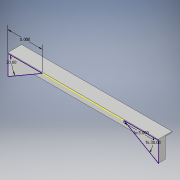
# Autodesk Inventor part: Wire Housing Lid vglue
Saved by Autodesk Inventor 2019 (Build 230136000, 136)
## iProperties
Created: 2020-03-05
Part Number: Wire Housing Lid vglue
Material: Generic
Document SubType Name: Modeling
Designer: Obscure_Decision
Density: 1 g/cm^3
Appearance: Default
Author: Obscure_Decision
Autodesk Inventor part; units mm, degrees
ref_plane "YZ Plane" through (0, 0, 0) normal (1, 0, 0) x (0, 1, 0)
ref_plane "XZ Plane" through (0, 0, 0) normal (0, 1, 0) x (-1, 0, 0)
ref_plane "XY Plane" through (0, 0, 0) normal (0, 0, 1) x (1, 0, 0)
sketch "Sketch1" plane through (0, 0, 0) normal (0, 1, 0) x (-1, 0, 0)
  line L0 (277.6855, 25.4) -> (-277.6855, 25.4)
  line L1 (-277.6855, 25.4) -> (-277.6855, -25.4)
  line L2 (-277.6855, -25.4) -> (277.6855, -25.4)
  line L3 (277.6855, -25.4) -> (277.6855, 25.4)
  line L4 (277.6855, 25.4) -> (-277.6855, -25.4) construction
  line L5 (-277.6855, 25.4) -> (277.6855, -25.4) construction
  point P0 (0, 0)
  dimension "d0" = 555.371
  dimension "d1" = 50.8
  constraints: 12 end point, 2 midpoint, 2 parallel, 1 horizontal, 1 perpendicular
  measures "d0" distance of L2.end L1.end
  measures "d1" distance of L1.end L0.end
extrude "Extrusion1" add sketch "Sketch1" along normal blind 3.048
sketch "Sketch2" plane through (-277.6855, 0, 25.4) normal (0, 0, 1) x (1, 0, 0)
  line L0 (0, 0) -> (555.371, 0) projected
  line L1 (555.371, 0) -> (428.371, 0)
  line L2 (555.371, 0) -> (555.371, -73.3235)
  line L3 (555.371, -73.3235) -> (428.371, 0)
  line L4 (0, 0) -> (127, 0)
  line L5 (127, 0) -> (0, -73.3235)
  line L6 (0, -73.3235) -> (0, 0)
  point P0 (277.6855, 0)
  dimension "d6" = 127
  dimension "d8" = 127
  dimension "d9" = 30
  dimension "d15" = 30
  constraints: 12 end point, 2 point on line, 1 perpendicular, 1 vertical
  measures "d6" distance of L0.end L1.end
  measures "d8" distance of L0.start L4.end
  measures "d9" angle of L4 L5
  measures "d15" angle of L0 L3
extrude "Extrusion2" add sketch "Sketch2" against normal blind 25.4 contours L0 L2 L3
extrude "Extrusion3" add sketch "Sketch2" against normal blind 25.4 contours L0 L5 L6
sketch "Sketch3" plane through (0, 0, 0) normal (0, -1, 0) x (1, 0, 0)
  line L0 (-277.6855, 25.4) -> (277.6855, 25.4) construction
  line L1 (-277.6855, 25.4) -> (0, 25.4) construction
  line L2 (0, 0) -> (0, 25.4) construction
  line L3 (184.15, 25.4) -> (-184.15, 25.4)
  line L4 (-184.15, 25.4) -> (-184.15, 0)
  line L5 (-184.15, 0) -> (184.15, 0)
  line L6 (184.15, 0) -> (184.15, 25.4)
  line L7 (184.15, 25.4) -> (-184.15, 0) construction
  line L8 (-184.15, 25.4) -> (184.15, 0) construction
  point P0 (0, 12.7)
  dimension "d16" = 368.3
  constraints: 16 end point, 4 midpoint, 2 parallel, 2 perpendicular, 1 horizontal
  measures "d16" distance of L5.end L4.end
extrude "Extrusion4" add sketch "Sketch3" along normal blind 19.05
equation "\"d6\" = d8"
equation "\"d15\" = d9"
body "Solid1"
